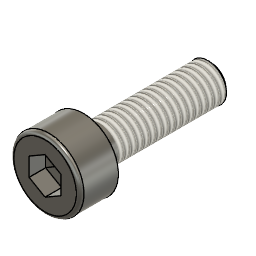
Space Maus V1 (Autodesk Fusion 360 archive; units mm, degrees)
design "Innensechskantschraube DIN 912 - M3 x 0.5 x 10 Stahl 4.6 Einfach"
description: Innensechskantschraube DIN 912 - M3 x 0.5 x 10
part number: DIN 912 - M3 x 0.5 x 10 Stahl 4.6 Einfach
Autodesk Fusion 360 part; units mm, degrees
sketch "Sketch1" plane through (0, 0, 0) normal (0, 1, 0) x (1, 0, 0)
  line L0 (-1.5, 0) -> (-1.5, 10)
  line L1 (-1.5, 10) -> (0, 10)
  line L2 (0, 10) -> (0, -3)
  line L3 (-1.5, 0) -> (-2.75, 0)
  line L4 (-2.75, 0) -> (-2.75, -3)
  line L5 (-2.75, -3) -> (0, -3)
  dimension "d101" = 10
  dimension "d102" = 3
  dimension "d109" = 5.5
  dimension "d110" = 3
  constraint perpendicular L0 L1
  constraint collinear origin L1.end L2.end
  constraint perpendicular L0 L3
  constraint coincident origin L3
  constraint vertical L2
  constraint coincident L2 L5.end
  constraint perpendicular L2 L5
  measures "d101" distance of origin L1
  measures "d102" distance of L3.end L5
revolve "Revolve1" add sketch "Sketch1" angle 360 about axis through (0, 0, -10) along (0, 0, 1)
ref_plane "WorkPlane1" through (0, 0, 3) normal (0, 0, 1) x (1, 0, 0)
sketch "Sketch6" plane through (0, 0, 3) normal (0, 0, 1) x (1, 0, 0)
  line L0 (0, -1.4434) -> (1.25, -0.7217)
  line L1 (1.25, -0.7217) -> (1.25, 0.7217)
  line L2 (1.25, 0.7217) -> (0, 1.4434)
  line L3 (0, 1.4434) -> (-1.25, 0.7217)
  line L4 (-1.25, 0.7217) -> (-1.25, -0.7217)
  line L5 (-1.25, -0.7217) -> (0, -1.4434)
  dimension "d111" = 2.5
  constraint vertical L1
  measures "d111" distance of L1 L4
extrude "Extrude1" cut sketch "Sketch6" against normal blind 1.3
extrude "Extrude2" cut 1 faces at (0.4167, -0.2406, 1.7) along direction (0, 0, -1) blind 1.3 draft -85
thread "Thread3" "ISO Metric profile 3.0 M3x0.5 M3x0.5 6g" major diameter 2.927 minor diameter 2.3555 pitch 0.5 angle 60 resizes the face on face at (-1.4981, 0.0748, -6.6667) from (0, 0, -1.25) to (0, 0, -10)
fillet "Fillet4" radius 0.3 1 edges at (-2.5639, 0.9944, 3)
sketch "Sketch7" plane through (0, 0, 0) normal (0, 1, 0) x (1, 0, 0)
  line L0 (-1.53, 10) -> (-1.53, 9.6933)
  line L1 (-1.53, 9.6933) -> (-1.1933, 10)
  line L2 (0, 10) -> (0, -3)
  line L3 (-1.53, 10) -> (0, 10)
  dimension "d104" = 1.1933
  dimension "d105" = 1.53
  dimension "d106" = 0.3067
  constraint coincident L2.start L3.end
  constraint perpendicular L2 L3
  constraint coincident L1.end L3
  constraint perpendicular L0 L3
  measures "d104" distance of L1.end L2
  measures "d105" distance of L0 L2.start
  measures "d106" distance of L0.end L3
revolve "Revolve3" cut sketch "Sketch7" angle 360 about axis through (0, 0, 1.75) along (0, 0, 1)
equation "adsk_nomlen = 10.00 mm"
equation "adsk_headh = 3.00 mm"
equation "adsk_headdia = 5.50 mm"
equation "adsk_nomdia = 3.00 mm"
equation "adsk_philwidth = 2.50 mm"
equation "d31 = -adsk_phildepth"
equation "adsk_phildepth = 1.30 mm"
equation "d71 = adsk_headh"
equation "d76 = -adsk_phildepth"
equation "adsk_thrlen = 8.75 mm"
equation "d86 = adsk_nomdia * 0.1"
equation "adsk_startlen = 0.306725 mm"
equation "adsk_endpointdia = 2.38655 mm"
equation "d101 = adsk_nomlen"
equation "d102 = adsk_headh"
equation "d104 = adsk_endpointdia / 2"
equation "d105 = adsk_nomdia * 0.51"
equation "d106 = adsk_startlen"
equation "d108 = min(adsk_thrlen; adsk_nomlen - 0.001 mm)"
equation "d109 = adsk_headdia"
equation "d110 = adsk_nomdia"
equation "d111 = adsk_philwidth"

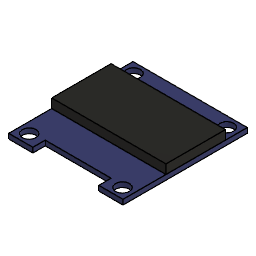
design "Screen"
Autodesk Fusion 360 part; units mm, degrees
sketch "Skizze1" plane through (0, 0, 0) normal (0, 0, 1) x (1, 0, 0) in component "board"
  line L0 (0, 0) -> (0, 67.6805) construction
  line L1 (0, 27.2) -> (-12.5, 27.2)
  line L2 (-12.5, 27.2) -> (-12.5, 0)
  line L3 (-12.5, 0) -> (-7.2, 0)
  line L4 (-7.2, 0) -> (-7.2, 2.7)
  line L5 (-7.2, 2.7) -> (0, 2.7)
  circle A0 centre (-10.2, 25) radius 1.5
  circle A1 centre (-10.2, 2.2) radius 1.5
  line L6 (12.5, 27.2) -> (12.5, 0)
  circle A2 centre (10.2, 25) radius 1.5
  circle A3 centre (10.2, 2.2) radius 1.5
  line L7 (12.5, 0) -> (7.2, 0)
  line L8 (7.2, 0) -> (7.2, 2.7)
  line L9 (7.2, 2.7) -> (0, 2.7)
  line L10 (0, 27.2) -> (12.5, 27.2)
  dimension "d1" = 12.5
  dimension "d2" = 27.2
  dimension "d3" = 5.3
  dimension "d4" = 2.7
  dimension "d5" = 3
  dimension "d6" = 2.2
  dimension "d7" = 2.3
  dimension "d8" = 3
  dimension "d9" = 2.3
  dimension "d10" = 2.2
  constraint coincident L0.start origin
  constraint vertical L0
  constraint coincident L0 L1.start
  constraint perpendicular L0 L1
  constraint perpendicular L1 L2
  constraint perpendicular L2 L3
  constraint perpendicular L1 L4
  constraint coincident L0 L5.end
  constraint perpendicular L0 L5
  constraint coincident L0.start L3
  constraint symmetric L0 L1.start L10.start
  constraint symmetric L0 L1.end L6.start
  constraint symmetric L0 L2.end L6.end
  constraint symmetric L0 L3.end L7.end
  constraint symmetric L0 L4.end L8.end
  constraint symmetric L0 L5.end L9.end
  constraint symmetric L0 A0 A2
  constraint symmetric L0 A1 A3
  measures "d1" distance of L1.start L1.end
  measures "d2" distance of L1.end L2.end
  measures "d3" distance of L2.end L3.end
  measures "d4" distance of L3.end L4.end
  measures "d5" diameter of A0
  measures "d6" distance of L1 A0.centre
  measures "d7" distance of L2 A0.centre
  measures "d8" diameter of A1
  measures "d9" distance of L2 A1.centre
  measures "d10" distance of L3 A1.centre
  measures "d13" distance of L7.end
extrude "Extrusion1" add sketch "Skizze1" along normal blind 1.1 makes body 1 in component "board"
sketch "Skizze1 (2)" plane through (0, 0, 1.1) normal (0, 0, 1) x (-1, 0, 0) in component "Component"
  circle A0 centre (-10.2, -2.2) radius 1.5
  circle A1 centre (10.2, -25) radius 1.5
  circle A2 centre (-10.2, -25) radius 1.5
  circle A3 centre (10.2, -2.2) radius 1.5
  line L0 (12.5, -27.2) -> (12.5, 0)
  line L1 (12.5, 0) -> (7.2, 0)
  line L2 (7.2, 0) -> (7.2, -2.7)
  line L3 (7.2, -2.7) -> (-7.2, -2.7)
  line L4 (-7.2, -2.7) -> (-7.2, 0)
  line L5 (-7.2, 0) -> (-12.5, 0)
  line L6 (-12.5, 0) -> (-12.5, -27.2)
  line L7 (-12.5, -27.2) -> (12.5, -27.2)
  line L8 (12.5, -22.4) -> (-12.5, -22.4)
  line L9 (-12.5, -22.4) -> (-12.5, -9.4)
  line L10 (-12.5, -9.4) -> (12.5, -9.4)
  line L11 (12.5, -9.4) -> (12.5, -22.4)
  dimension "d13" = 13
  dimension "d14" = 4.8
  constraint horizontal L8
  constraint vertical L9
  constraint horizontal L10
  constraint vertical L11
  constraint coincident L6 L9.end
  constraint coincident L0 L8.start
  measures "d13" distance of L8.start L10.end
  measures "d14" distance of L7 L8
extrude "Extrusion1'" add sketch "Skizze1 (2)" along normal blind 2 separate body contours L0 L6 L8 L9 L10 L11 makes body 2 in component "Component"
component "board" placed x (1, 0, 0) y (0, 1, 0) z (0, 0, 1) at (0, 0, 0)
component "Component" placed x (1, 0, 0) y (0, 1, 0) z (0, 0, 1) at (0, 0, 0)
equation "d1 = ( 25 / 2 ) * 1 mm"
equation "d6 = d5 / 2 + 0.7 mm"
equation "d7 = d5 / 2 + 0.8 mm"
equation "d9 = d7"
equation "d10 = d6"

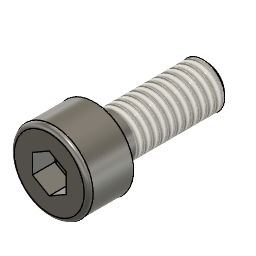
design "Innensechskantschraube DIN 912 - M4 x 0.7 x 10 Stahl 4.6 Einfach"
description: Innensechskantschraube DIN 912 - M4 x 0.7 x 10
part number: DIN 912 - M4 x 0.7 x 10 Stahl 4.6 Einfach
Autodesk Fusion 360 part; units mm, degrees
sketch "Sketch1" plane through (0, 0, 0) normal (0, 1, 0) x (1, 0, 0)
  line L0 (-2, 0) -> (-2, 10)
  line L1 (-2, 10) -> (0, 10)
  line L2 (0, 10) -> (0, -4)
  line L3 (-2, 0) -> (-3.5, 0)
  line L4 (-3.5, 0) -> (-3.5, -4)
  line L5 (-3.5, -4) -> (0, -4)
  dimension "d101" = 10
  dimension "d102" = 4
  dimension "d109" = 7
  dimension "d110" = 4
  constraint perpendicular L0 L1
  constraint collinear origin L1.end L2.end
  constraint perpendicular L0 L3
  constraint coincident origin L3
  constraint vertical L2
  constraint coincident L2 L5.end
  constraint perpendicular L2 L5
  measures "d101" distance of origin L1
  measures "d102" distance of L3.end L5
revolve "Revolve1" add sketch "Sketch1" angle 360 about axis through (0, 0, -10) along (0, 0, 1)
ref_plane "WorkPlane1" through (0, 0, 4) normal (0, 0, 1) x (1, 0, 0)
sketch "Sketch6" plane through (0, 0, 4) normal (0, 0, 1) x (1, 0, 0)
  line L0 (0, -1.7321) -> (1.5, -0.866)
  line L1 (1.5, -0.866) -> (1.5, 0.866)
  line L2 (1.5, 0.866) -> (0, 1.7321)
  line L3 (0, 1.7321) -> (-1.5, 0.866)
  line L4 (-1.5, 0.866) -> (-1.5, -0.866)
  line L5 (-1.5, -0.866) -> (0, -1.7321)
  dimension "d111" = 3
  constraint vertical L1
  measures "d111" distance of L1 L4
extrude "Extrude1" cut sketch "Sketch6" against normal blind 2
extrude "Extrude2" cut 1 faces at (0, -0.5774, 2) along direction (0, 0, -1) blind 2 draft -85
thread "Thread3" "ISO Metric profile 4.0 M4x0.7 M4x0.7 6g" major diameter 3.908 minor diameter 3.111 pitch 0.7 angle 60 resizes the face on face at (-1.9975, 0.0997, -6.6667) from (0, 0, -1.75) to (0, 0, -10)
fillet "Fillet4" radius 0.4 1 edges at (-3.2631, 1.2657, 4)
sketch "Sketch7" plane through (0, 0, 0) normal (0, 1, 0) x (1, 0, 0)
  line L0 (-2.04, 10) -> (-2.04, 9.5706)
  line L1 (-2.04, 9.5706) -> (-1.5706, 10)
  line L2 (0, 10) -> (0, -4)
  line L3 (-2.04, 10) -> (0, 10)
  dimension "d104" = 1.5706
  dimension "d105" = 2.04
  dimension "d106" = 0.4294
  constraint coincident L2.start L3.end
  constraint perpendicular L2 L3
  constraint coincident L1.end L3
  constraint perpendicular L0 L3
  measures "d104" distance of L1.end L2
  measures "d105" distance of L0 L2.start
  measures "d106" distance of L0.end L3
revolve "Revolve3" cut sketch "Sketch7" angle 360 about axis through (0, 0, 1.75) along (0, 0, 1)
equation "adsk_nomlen = 10.00 mm"
equation "adsk_headh = 4.00 mm"
equation "adsk_headdia = 7.00 mm"
equation "adsk_nomdia = 4.00 mm"
equation "adsk_philwidth = 3.00 mm"
equation "d31 = -adsk_phildepth"
equation "adsk_phildepth = 2.00 mm"
equation "d71 = adsk_headh"
equation "d76 = -adsk_phildepth"
equation "adsk_thrlen = 8.25 mm"
equation "d86 = adsk_nomdia * 0.1"
equation "adsk_startlen = 0.429415 mm"
equation "adsk_endpointdia = 3.14117 mm"
equation "d101 = adsk_nomlen"
equation "d102 = adsk_headh"
equation "d104 = adsk_endpointdia / 2"
equation "d105 = adsk_nomdia * 0.51"
equation "d106 = adsk_startlen"
equation "d108 = min(adsk_thrlen; adsk_nomlen - 0.001 mm)"
equation "d109 = adsk_headdia"
equation "d110 = adsk_nomdia"
equation "d111 = adsk_philwidth"

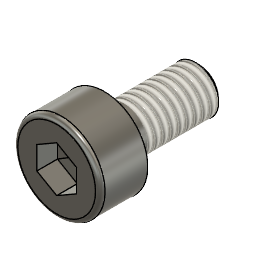
design "Innensechskantschraube DIN 912 - M3 x 0.5 x 6 Stahl 4.6 Einfach"
description: Innensechskantschraube DIN 912 - M3 x 0.5 x 6
part number: DIN 912 - M3 x 0.5 x 6 Stahl 4.6 Einfach
Autodesk Fusion 360 part; units mm, degrees
sketch "Sketch1" plane through (0, 0, 0) normal (0, 1, 0) x (1, 0, 0)
  line L0 (-1.5, 0) -> (-1.5, 6)
  line L1 (-1.5, 6) -> (0, 6)
  line L2 (0, 6) -> (0, -3)
  line L3 (-1.5, 0) -> (-2.75, 0)
  line L4 (-2.75, 0) -> (-2.75, -3)
  line L5 (-2.75, -3) -> (0, -3)
  dimension "d101" = 6
  dimension "d102" = 3
  dimension "d109" = 5.5
  dimension "d110" = 3
  constraint perpendicular L0 L1
  constraint collinear origin L1.end L2.end
  constraint perpendicular L0 L3
  constraint coincident origin L3
  constraint vertical L2
  constraint coincident L2 L5.end
  constraint perpendicular L2 L5
  measures "d101" distance of origin L1
  measures "d102" distance of L3.end L5
revolve "Revolve1" add sketch "Sketch1" angle 360 about axis through (0, 0, -6) along (0, 0, 1)
ref_plane "WorkPlane1" through (0, 0, 3) normal (0, 0, 1) x (1, 0, 0)
sketch "Sketch6" plane through (0, 0, 3) normal (0, 0, 1) x (1, 0, 0)
  line L0 (0, -1.4434) -> (1.25, -0.7217)
  line L1 (1.25, -0.7217) -> (1.25, 0.7217)
  line L2 (1.25, 0.7217) -> (0, 1.4434)
  line L3 (0, 1.4434) -> (-1.25, 0.7217)
  line L4 (-1.25, 0.7217) -> (-1.25, -0.7217)
  line L5 (-1.25, -0.7217) -> (0, -1.4434)
  dimension "d111" = 2.5
  constraint vertical L1
  measures "d111" distance of L1 L4
extrude "Extrude1" cut sketch "Sketch6" against normal blind 1.3
extrude "Extrude2" cut 1 faces at (0.4167, -0.2406, 1.7) along direction (0, 0, -1) blind 1.3 draft -85
thread "Thread3" "ISO Metric profile 3.0 M3x0.5 M3x0.5 6g" major diameter 2.927 minor diameter 2.3555 pitch 0.5 angle 60 resizes the face on face at (-1.4925, 0.1494, -4) from (0, 0, -1.25) to (0, 0, -6)
fillet "Fillet4" radius 0.3 1 edges at (-2.5639, 0.9944, 3)
sketch "Sketch7" plane through (0, 0, 0) normal (0, 1, 0) x (1, 0, 0)
  line L0 (-1.53, 6) -> (-1.53, 5.6933)
  line L1 (-1.53, 5.6933) -> (-1.1933, 6)
  line L2 (0, 6) -> (0, -3)
  line L3 (-1.53, 6) -> (0, 6)
  dimension "d104" = 1.1933
  dimension "d105" = 1.53
  dimension "d106" = 0.3067
  constraint coincident L2.start L3.end
  constraint perpendicular L2 L3
  constraint coincident L1.end L3
  constraint perpendicular L0 L3
  measures "d104" distance of L1.end L2
  measures "d105" distance of L0 L2.start
  measures "d106" distance of L0.end L3
revolve "Revolve3" cut sketch "Sketch7" angle 360 about axis through (0, 0, 1.75) along (0, 0, 1)
equation "adsk_nomlen = 6.00 mm"
equation "adsk_headh = 3.00 mm"
equation "adsk_headdia = 5.50 mm"
equation "adsk_nomdia = 3.00 mm"
equation "adsk_philwidth = 2.50 mm"
equation "d31 = -adsk_phildepth"
equation "adsk_phildepth = 1.30 mm"
equation "d71 = adsk_headh"
equation "d76 = -adsk_phildepth"
equation "adsk_thrlen = 4.75 mm"
equation "d86 = adsk_nomdia * 0.1"
equation "adsk_startlen = 0.306725 mm"
equation "adsk_endpointdia = 2.38655 mm"
equation "d101 = adsk_nomlen"
equation "d102 = adsk_headh"
equation "d104 = adsk_endpointdia / 2"
equation "d105 = adsk_nomdia * 0.51"
equation "d106 = adsk_startlen"
equation "d108 = min(adsk_thrlen; adsk_nomlen - 0.001 mm)"
equation "d109 = adsk_headdia"
equation "d110 = adsk_nomdia"
equation "d111 = adsk_philwidth"

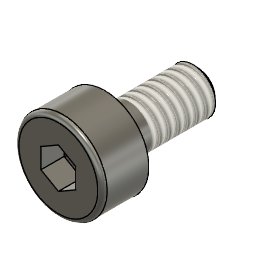
design "Zylinderschraube mit gestanztem Innensechskant ANSI B18.3.1M - M2x0.4 x 4 Stahlklasse 2 Einfach"
description: Zylinderschraube mit gestanztem Innensechskant ANSI B18.3.1M - M2x0.4 x 4
part number: BSHCS ANSI B18.3.1M - M2x0.4 x 4 Stahlklasse 2 Einfach
Autodesk Fusion 360 part; units mm, degrees
sketch "Sketch1" plane through (0, 0, 0) normal (0, 1, 0) x (1, 0, 0)
  line L0 (-1, 0) -> (-1, 4)
  line L1 (-1, 4) -> (0, 4)
  line L2 (0, 4) -> (0, -2)
  line L3 (-1, 0) -> (-1.9, 0)
  line L4 (-1.9, 0) -> (-1.9, -2)
  line L5 (-1.9, -2) -> (0, -2)
  dimension "d101" = 4
  dimension "d102" = 2
  dimension "d109" = 3.8
  dimension "d110" = 2
  constraint perpendicular L0 L1
  constraint collinear origin L1.end L2.end
  constraint perpendicular L0 L3
  constraint coincident origin L3
  constraint vertical L2
  constraint coincident L2 L5.end
  constraint perpendicular L2 L5
  measures "d101" distance of origin L1
  measures "d102" distance of L3.end L5
revolve "Revolve1" add sketch "Sketch1" angle 360 about axis through (0, 0, -4) along (0, 0, 1)
ref_plane "WorkPlane1" through (0, 0, 2) normal (0, 0, 1) x (1, 0, 0)
sketch "Sketch6" plane through (0, 0, 2) normal (0, 0, 1) x (1, 0, 0)
  line L0 (0, -0.866) -> (0.75, -0.433)
  line L1 (0.75, -0.433) -> (0.75, 0.433)
  line L2 (0.75, 0.433) -> (0, 0.866)
  line L3 (0, 0.866) -> (-0.75, 0.433)
  line L4 (-0.75, 0.433) -> (-0.75, -0.433)
  line L5 (-0.75, -0.433) -> (0, -0.866)
  dimension "d111" = 1.5
  constraint vertical L1
  measures "d111" distance of L1 L4
extrude "Extrude1" cut sketch "Sketch6" against normal blind 1
extrude "Extrude2" cut 1 faces at (0, -0.2887, 1) along direction (0, 0, -1) blind 1 draft -85
thread "Thread3" "ANSI Metric M Profile 2.0 M2x0.4 M2x0.4 4g6g" major diameter 1.9335 minor diameter 1.4905 pitch 0.4 angle 60 resizes the face on face at (-0.995, 0.0996, -2.6667) from (0, 0, -1.0454) to (0, 0, -4)
fillet "Fillet4" radius 0.2 1 edges at (-1.7714, 0.6871, 2)
sketch "Sketch7" plane through (0, 0, 0) normal (0, 1, 0) x (1, 0, 0)
  line L0 (-1.02, 4) -> (-1.02, 3.7546)
  line L1 (-1.02, 3.7546) -> (-0.7546, 4)
  line L2 (0, 4) -> (0, -2)
  line L3 (-1.02, 4) -> (0, 4)
  dimension "d104" = 0.7546
  dimension "d105" = 1.02
  dimension "d106" = 0.2454
  constraint coincident L2.start L3.end
  constraint perpendicular L2 L3
  constraint coincident L1.end L3
  constraint perpendicular L0 L3
  measures "d104" distance of L1.end L2
  measures "d105" distance of L0 L2.start
  measures "d106" distance of L0.end L3
revolve "Revolve3" cut sketch "Sketch7" angle 360 about axis through (0, 0, 1.75) along (0, 0, 1)
equation "adsk_nomlen = 4.00 mm"
equation "adsk_headh = 2.00 mm"
equation "adsk_headdia = 3.80 mm"
equation "adsk_nomdia = 2.00 mm"
equation "adsk_philwidth = 1.50 mm"
equation "d31 = -adsk_phildepth"
equation "adsk_phildepth = 1.00 mm"
equation "d71 = adsk_headh"
equation "d76 = -adsk_phildepth"
equation "adsk_thrlen = 2.95462 mm"
equation "d86 = adsk_nomdia * 0.1"
equation "adsk_startlen = 0.24538 mm"
equation "adsk_endpointdia = 1.50924 mm"
equation "d101 = adsk_nomlen"
equation "d102 = adsk_headh"
equation "d104 = adsk_endpointdia / 2"
equation "d105 = adsk_nomdia * 0.51"
equation "d106 = adsk_startlen"
equation "d108 = min(adsk_thrlen; adsk_nomlen - 0.001 mm)"
equation "d109 = adsk_headdia"
equation "d110 = adsk_nomdia"
equation "d111 = adsk_philwidth"
